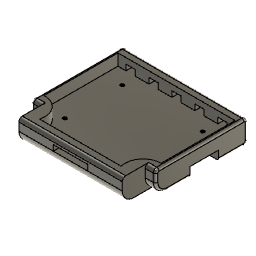
Carcasa Muñeca v2.2 (Autodesk Fusion 360 design; units mm, degrees)
Autodesk Fusion 360 part; units mm, degrees
sketch "Sketch10" plane through (0, 0, 0) normal (0, 0, 1) x (1, 0, 0)
  line L0 (0, -50) -> (0, 50) construction
  line L1 (0, 50) -> (-57, 50)
  line L2 (-57, 50) -> (-57, 0)
  line L3 (0, -50) -> (-45, -50)
  line L4 (-45, -50) -> (-45, -30)
  arc A0 (-57, 0) -> (-45, -30) centre (-7.0663, 2.5735) ccw
  line L5 (0, -50) -> (45, -50)
  line L6 (45, -50) -> (45, -30)
  arc A1 (45, -30) -> (57, 0) centre (7.0663, 2.5735) ccw
  line L7 (57, 50) -> (57, 0)
  line L8 (0, 50) -> (57, 50)
  dimension "d19" = 100
  dimension "d20" = 57
  dimension "d21" = 50
  dimension "d22" = 45
  dimension "d23" = 20
  dimension "d24" = 50
  dimension "d25" = 30
  constraint vertical L0
  constraint midpoint L0 origin
  constraint perpendicular L0 L1
  constraint perpendicular L1 L2
  constraint perpendicular L0 L3
  constraint perpendicular L3 L4
  constraint symmetric L3.start L0 L5.start
  constraint symmetric L1.start L0 L8.start
  constraint symmetric L0 L1.end L7.start
  constraint symmetric L0 L2.end A1.end
  constraint symmetric L0 L3.end L5.end
  constraint symmetric L0 L4.end L6.end
  constraint symmetric L0 A0 A1
  measures "d19" distance of L0.start L0.end
  measures "d20" distance of L0.end L1.end
  measures "d21" distance of L1.end L2.end
  measures "d22" distance of L0.start L3.end
  measures "d23" distance of L3.end L4.end
  measures "d24" radius of A0
  measures "d25" vertical distance of L2.end L4.end
sketch "Sketch12" plane through (0, 0, 0) normal (1, 0, 0) x (0, 1, 0)
  line L0 (0, 10) -> (0, -10) construction
  line L1 (0, 10) -> (47, 10)
  line L2 (50, 7) -> (50, -7)
  line L3 (47, -10) -> (0, -10)
  arc A0 (50, 7) -> (47, 10) centre (47, 7) ccw
  line L4 (0, 10) -> (-47, 10)
  line L5 (-50, 7) -> (-50, 0)
  line L6 (-40, -10) -> (0, -10)
  arc A1 (-47, 10) -> (-50, 7) centre (-47, 7) ccw
  arc A2 (-50, 0) -> (-40, -10) centre (-40, 0) ccw
  arc A3 (47, -10) -> (50, -7) centre (47, -7) ccw
  dimension "d30" = 3
  dimension "d31" = 47
  dimension "d34" = 3
  dimension "d35" = 10
  dimension "d36" = 7
  dimension "d37" = 40
  dimension "d38" = 3
  dimension "d39" = 47
  dimension "d40" = 14
  constraint vertical L0
  constraint midpoint L0 origin
  constraint perpendicular L0 L1
  constraint perpendicular L1 L2
  constraint tangent L1 A0
  constraint tangent L2 A0
  constraint perpendicular L0 L4
  constraint perpendicular L4 L5
  constraint tangent L5 A1
  constraint tangent L4 A1
  constraint tangent L6 A2
  constraint tangent L5 A2
  constraint tangent L3 A3
  constraint tangent L2 A3
  measures "d30" radius of A0
  measures "d31" distance of L0.start L1.end
  measures "d34" radius of A1
  measures "d35" radius of A2
  measures "d36" distance of L5.start L5.end
  measures "d37" distance of L0.end L6.start
  measures "d38" radius of A3
  measures "d39" distance of L0.end L3.start
  measures "d40" distance of L2.start L2.end
extrude "Extrude1" add sketch "Sketch12" along normal mid plane 90 makes body 1
ref_plane "PlanoDeObra18" through (-54, 0, 0) normal (-1, 0, 0) x (0, -1, 0)
sketch "Boceto31" plane through (-45, 0, 0) normal (-1, 0, 0) x (0, -1, 0)
  line L0 (47, 10) -> (-47, 10)
  arc A0 (-47, 10) -> (-50, 7) centre (-47, 7) ccw
  line L1 (-50, 7) -> (-50, -7)
  arc A1 (-50, -7) -> (-47, -10) centre (-47, -7) ccw
  line L2 (-47, -10) -> (0, -10)
  line L3 (0, -10) -> (40, -10)
  arc A2 (40, -10) -> (50, 0) centre (40, 0) ccw
  line L4 (50, 0) -> (50, 7)
  arc A3 (50, 7) -> (47, 10) centre (47, 7) ccw
  arc A4 (-50, -7) -> (-47, -10) centre (-47, -7) ccw
  line L5 (-47, -7) -> (-50, -7) construction
  line L6 (-47, -7) -> (-47, -10) construction
  line L7 (-47, -10) -> (20, -10)
  line L8 (-47, 10) -> (27, 10)
  line L9 (-50, 7) -> (-50, -7)
  arc A5 (30, 7) -> (26.9876, 10) centre (27, 7) ccw
  line L10 (27, 7) -> (30, 7) construction
  line L11 (27, 7) -> (26.9876, 10) construction
  arc A6 (20, -10) -> (30, 0) centre (20, 0) ccw
  line L12 (20, 0) -> (20, -10) construction
  line L13 (20, 0) -> (30, 0) construction
  line L14 (30, 0) -> (30, 7)
  dimension "d172" = 3
  dimension "d174" = 67
  dimension "d175" = 74
  dimension "d176" = 3
  dimension "d178" = 10
  constraint coincident A1.centre A4.centre
  constraint coincident A1.end L2.start
  constraint perpendicular L6 L7
  constraint coincident L0.end A0.start
  constraint parallel L0 L8
  constraint coincident A0.end L1.start
  constraint tangent A4 L9
  constraint tangent L8 A5
  constraint tangent L7 A6
  constraint tangent A6 L14
  constraint tangent A5 L14
  constraint perpendicular L8 L14
  measures "d172" radius of A4
  measures "d174" distance of A1.end L7.end
  measures "d175" distance of L0.end L8.end
  measures "d176" radius of A5
  measures "d178" radius of A6
extrude "Extruir14" add sketch "Boceto31" along normal blind 9 contours L0 A0 L1 A1 L2 L3 A4 L7 L8 L9 A5 A6 L14 bodies 1
sketch "Boceto32" plane through (45, 0, 0) normal (1, 0, 0) x (0, 1, 0)
  line L0 (47, 10) -> (-47, 10)
  arc A0 (-47, 10) -> (-50, 7) centre (-47, 7) ccw
  line L1 (-50, 7) -> (-50, 0)
  arc A1 (-50, 0) -> (-40, -10) centre (-40, 0) ccw
  line L2 (-40, -10) -> (0, -10)
  line L3 (0, -10) -> (47, -10)
  arc A2 (47, -10) -> (50, -7) centre (47, -7) ccw
  line L4 (50, -7) -> (50, 7)
  arc A3 (50, 7) -> (47, 10) centre (47, 7) ccw
  arc A4 (50, 7) -> (47, 10) centre (47, 7) ccw
  line L5 (47, 7) -> (50, 7) construction
  line L6 (47, 7) -> (47, 10) construction
  line L7 (47, 10) -> (-27, 10)
  arc A5 (47, -10) -> (50, -7) centre (47, -7) ccw
  line L8 (47, -7) -> (47, -10) construction
  line L9 (47, -7) -> (50, -7) construction
  line L10 (50, 7) -> (50, -7)
  line L11 (47, -10) -> (-20, -10)
  arc A6 (-30, 0) -> (-20, -10) centre (-20, 0) ccw
  line L12 (-20, 0) -> (-30, 0) construction
  line L13 (-20, 0) -> (-20, -10) construction
  arc A7 (-27, 10) -> (-30, 7) centre (-27, 7) ccw
  line L14 (-27, 7) -> (-27, 10) construction
  line L15 (-27, 7) -> (-30, 7) construction
  line L16 (-30, 7) -> (-30, 0)
  dimension "d182" = 3
  dimension "d184" = 74
  dimension "d185" = 3
  dimension "d187" = 67
  dimension "d188" = 10
  dimension "d190" = 3
  constraint coincident A3.centre A4.centre
  constraint coincident L0.start A3.end
  constraint perpendicular L6 L7
  constraint coincident A2.centre A5.centre
  constraint coincident L3.end A2.start
  constraint tangent A2 L10
  constraint perpendicular L10 L11
  constraint tangent A6 L16
  constraint tangent L7 A7
  constraint tangent L11 A6
  constraint tangent A5 L11
  constraint perpendicular L7 L16
  measures "d182" radius of A4
  measures "d184" distance of L0.start L7.end
  measures "d185" radius of A5
  measures "d187" distance of L3.end L11.end
  measures "d188" radius of A6
  measures "d190" radius of A7
extrude "Extruir15" add sketch "Boceto32" along normal blind 9 contours L0 L2 L3 A2 L4 A3 A4 L7 A5 L10 L11 A6 A7 L16 bodies 1
ref_plane "PlanoDeObra19" through (0, 0, 0) normal (0, 0, 1) x (0, -1, 0)
sketch "Boceto33" plane through (0, 0, 0) normal (0, 0, 1) x (1, 0, 0)
  line L0 (-43.8537, 42.0783) -> (51, 42.2395)
  line L1 (51, 42.2395) -> (-51, 42.2395)
  line L2 (-51, 42.2395) -> (-51, -22.125)
  line L3 (51, -22.125) -> (51, 42.2395)
  line L4 (-35.1587, -41.7605) -> (35.8108, -41.7605)
  arc A0 (-35.1587, -41.7605) -> (-51, -22.125) centre (-50.3046, -37.7717) ccw
  arc A1 (51, -22.125) -> (35.8108, -41.7605) centre (50.9606, -37.7871) ccw
  line L5 (0, 42.2395) -> (0.326, -41.7605)
  line L6 (54, -20) -> (54, 47)
  line L7 (-54, 47) -> (-54, -20)
  dimension "d202" = 84
  dimension "d256" = 3
  dimension "d257" = 3
  constraint horizontal L1
  constraint vertical L2
  constraint vertical L3
  constraint horizontal L4
  constraint equal L2 L3
  constraint equal A0 A1
  constraint midpoint L1 L5.start
  constraint midpoint L4 L5.end
  measures "d202" vertical distance of L5.start L5.end
  measures "d256" distance of L3 L6
  measures "d257" distance of L2 L7
extrude "Extruir16" cut sketch "Boceto33" along normal blind 10 bodies 1
ref_plane "PlanoDeObra20" through (54, 10, 10) normal (-1, 0, 0) x (0, -1, 0)
sketch "Boceto34" plane through (54, 10, 10) normal (-1, 0, 0) x (0, 0, -1)
  line L0 (20.0665, 10.0967) -> (12.0665, 10.0967)
  line L1 (12.0665, 10.0967) -> (12.0665, -14.9033)
  line L2 (12.0665, -14.9033) -> (20.0665, -14.9033)
  line L3 (20.0665, -14.9033) -> (20.0665, 10.0967)
  dimension "d205" = 8
  dimension "d206" = 25
  constraint horizontal L0
  constraint vertical L1
  constraint horizontal L2
  constraint vertical L3
  measures "d205" distance of L0.start L0.end
  measures "d206" distance of L0.start L2.end
extrude "Extruir17" cut sketch "Boceto34" along normal blind 15 bodies 1
ref_plane "PlanoDeObra21" through (46.5, -0.0967, -6.0333) normal (0, 1, 0) x (0, 0, -1)
sketch "Boceto35" plane through (46.5, -0.0967, -6.0333) normal (0, 1, 0) x (1, 0, 0)
  circle A0 centre (0, 0) radius 1.5
  dimension "d210" = 3
  constraint coincident A0.centre origin
  measures "d210" diameter of A0
extrude "Extruir18" add sketch "Boceto35" along normal up to surface (25 mm away) bodies 1
ref_plane "PlanoDeObra22" through (-54, 10, 0) normal (-1, 0, 0) x (0, -1, 0)
ref_plane "PlanoDeObra23" through (0, 50, 0) normal (0, 1, 0) x (0, 0, 1)
ref_plane "PlanoDeObra25" through (0, -50, 3.5) normal (0, -1, 0) x (0, 0, -1)
sketch "Boceto36" plane through (0, -50, 3.5) normal (0, -1, 0) x (1, 0, 0)
  line L0 (-15, 1.5) -> (15, 1.5)
  line L1 (15, 1.5) -> (15, -3.5)
  line L2 (15, -3.5) -> (-15, -3.5)
  line L3 (-15, -3.5) -> (-15, 1.5)
  line L4 (-15, 1.5) -> (15, -3.5) construction
  line L5 (15, 1.5) -> (-15, -3.5) construction
  point P0 (0, -1)
  dimension "d217" = 30
  dimension "d218" = 5
  constraint horizontal L0
  constraint perpendicular L0 L1
  constraint parallel L0 L2
  constraint parallel L1 L3
  constraint coincident L4 P0
  constraint coincident L5 P0
  measures "d217" distance of L1.end L2.end
  measures "d218" distance of L0.end L1.end
extrude "Extruir19" cut sketch "Boceto36" against normal blind 8.2397 bodies 1
fillet "Empalme5" radius 2 8 edges at (-54, 50, 0) (-54, 49.1213, -9.1213) (-54, 13.5, -10) (-54, -27.0711, -7.0711) (-54, -30, 3.5) (-54, -29.1213, 9.1213) (-54, 10, 10) (-54, 49.1213, 9.1213) on bodies 1
fillet "Empalme6" radius 2 9 edges at (54, 35.9516, -10) (54, 49.1213, -9.1213) (54, 50, 0) (54, 49.1213, 9.1213) (54, 10, 10) (54, -29.1213, 9.1213) (54, -30, 3.5) (54, -27.0711, -7.0711) (54, -10.0484, -10) on bodies 1
sketch "Boceto37" plane through (-54, 10, 0) normal (-1, 0, 0) x (0, 0, -1)
  line L0 (10.1981, 9.9042) -> (2.1981, 9.9042)
  line L1 (2.1981, 9.9042) -> (2.1981, -15.0958)
  line L2 (2.1981, -15.0958) -> (10.1981, -15.0958)
  line L3 (10.1981, -15.0958) -> (10.1981, 9.9042)
  dimension "d225" = 8
  dimension "d226" = 25
  constraint horizontal L0
  constraint vertical L1
  constraint horizontal L2
  constraint vertical L3
  measures "d225" distance of L0.start L0.end
  measures "d226" distance of L0.start L2.end
extrude "Extruir20" cut sketch "Boceto37" against normal blind 15 bodies 1
ref_plane "PlanoDeObra26" through (-46.5, 0.0958, -6.099) normal (0, 1, 0) x (0, 0, 1)
sketch "Boceto38" plane through (-46.5, 0.0958, -6.099) normal (0, 1, 0) x (1, 0, 0)
  circle A0 centre (0, 0) radius 1.5
  dimension "d233" = 3
  constraint coincident A0.centre origin
  measures "d233" diameter of A0
extrude "Extruir21" add sketch "Boceto38" along normal up to surface (25 mm away) bodies 1
sketch "Boceto39" plane through (0, 50, 0) normal (0, 1, 0) x (1, 0, 0)
  line L0 (44, 0) -> (36, 0)
  line L1 (36, 0) -> (36, -5)
  line L2 (36, -5) -> (44, -5)
  line L3 (44, -5) -> (44, 0)
  line L4 (52, 7) -> (52, -7)
  line L5 (24, 0) -> (16, 0)
  line L6 (16, 0) -> (16, -5)
  line L7 (16, -5) -> (24, -5)
  line L8 (24, -5) -> (24, 0)
  line L9 (4, 0) -> (-4, 0)
  line L10 (-4, 0) -> (-4, -5)
  line L11 (-4, -5) -> (4, -5)
  line L12 (4, -5) -> (4, 0)
  line L13 (11, -12) -> (-1, -12)
  line L14 (-16, 0) -> (-24, 0)
  line L15 (-24, 0) -> (-24, -5)
  line L16 (-24, -5) -> (-16, -5)
  line L17 (-16, -5) -> (-16, 0)
  line L18 (-36, 0) -> (-44, 0)
  line L19 (-44, 0) -> (-44, -5)
  line L20 (-44, -5) -> (-36, -5)
  line L21 (-36, -5) -> (-36, 0)
  line L22 (-52, -7) -> (-52, 7)
  dimension "d236" = 8
  dimension "d237" = 5
  dimension "d238" = 8
  dimension "d239" = 8
  dimension "d240" = 5
  dimension "d241" = 12
  dimension "d242" = 8
  dimension "d243" = 5
  dimension "d244" = 12
  dimension "d245" = 8
  dimension "d246" = 5
  dimension "d247" = 12
  dimension "d248" = 8
  dimension "d249" = 5
  dimension "d250" = 12
  dimension "d253" = 8
  constraint horizontal L0
  constraint vertical L1
  constraint horizontal L2
  constraint vertical L3
  constraint horizontal L5
  constraint vertical L6
  constraint horizontal L7
  constraint vertical L8
  constraint horizontal L9
  constraint vertical L10
  constraint horizontal L11
  constraint vertical L12
  constraint horizontal L13
  constraint horizontal L14
  constraint vertical L15
  constraint horizontal L16
  constraint vertical L17
  constraint horizontal L18
  constraint vertical L19
  constraint horizontal L20
  constraint vertical L21
  measures "d236" distance of L0.start L0.end
  measures "d237" distance of L0.start L2.end
  measures "d238" distance of L0.start L4
  measures "d239" distance of L5.start L5.end
  measures "d240" distance of L5.start L7.end
  measures "d241" distance of L0.end L5.start
  measures "d242" distance of L9.start L9.end
  measures "d243" distance of L9.start L11.end
  measures "d244" distance of L5.end L9.start
  measures "d245" distance of L14.start L14.end
  measures "d246" distance of L14.start L16.end
  measures "d247" distance of L9.end L14.start
  measures "d248" distance of L18.start L18.end
  measures "d249" distance of L18.start L20.end
  measures "d250" distance of L14.end L18.start
  measures "d253" distance of L18.end L22
extrude "Extruir22" cut sketch "Boceto39" against normal blind 8 bodies 1
sketch "Boceto40" plane through (0, 0, 0) normal (0, 0, 1) x (-1, 0, 0)
  line L0 (4, -42.2395) -> (16, -42.2395)
  line L1 (16, -42.2395) -> (16, -50)
  line L2 (16, -50) -> (24, -50)
  line L3 (24, -50) -> (24, -42.2395)
  line L4 (24, -42.2395) -> (36, -42.2395)
  line L5 (36, -42.2395) -> (36, -50)
  line L6 (36, -50) -> (44, -50)
  line L7 (44, -50) -> (44, -42.2395)
  line L8 (44, -42.2395) -> (51, -42.2395)
  line L9 (51, -42.2395) -> (51, 22.125)
  arc A0 (35.1587, 41.7605) -> (51, 22.125) centre (50.3046, 37.7717) ccw
  line L10 (35.1587, 41.7605) -> (15, 41.7605)
  line L11 (15, 41.7605) -> (15, 50)
  line L12 (15, 50) -> (-15, 50)
  line L13 (-15, 50) -> (-15, 41.7605)
  line L14 (-15, 41.7605) -> (-35.8108, 41.7605)
  arc A1 (-51, 22.125) -> (-35.8108, 41.7605) centre (-50.9606, 37.7871) ccw
  line L15 (-51, 22.125) -> (-51, -42.2395)
  line L16 (-51, -42.2395) -> (-44, -42.2395)
  line L17 (-44, -42.2395) -> (-44, -50)
  line L18 (-44, -50) -> (-36, -50)
  line L19 (-36, -50) -> (-36, -42.2395)
  line L20 (-36, -42.2395) -> (-24, -42.2395)
  line L21 (-24, -42.2395) -> (-24, -50)
  line L22 (-24, -50) -> (-16, -50)
  line L23 (-16, -50) -> (-16, -42.2395)
  line L24 (-16, -42.2395) -> (-4, -42.2395)
  line L25 (-4, -42.2395) -> (-4, -50)
  line L26 (-4, -50) -> (4, -50)
  line L27 (4, -50) -> (4, -42.2395)
sketch "Boceto41" plane through (0, 0, 0) normal (0, 0, 1) x (1, 0, 0)
  circle A0 centre (-35, 30) radius 1.525
  circle A1 centre (-35, -20) radius 1.525
  circle A2 centre (35, 30) radius 1.525
  circle A3 centre (35, -20) radius 1.525
  dimension "d260" = 3.05
  dimension "d261" = 3.05
  dimension "d262" = 3.05
  dimension "d264" = 70
  dimension "d265" = 50
  dimension "d266" = 3.05
  dimension "d267" = 70
  dimension "d268" = 50
  measures "d260" diameter of A0
  measures "d261" diameter of A1
  measures "d262" diameter of A2
  measures "d264" distance of A0.centre A2.centre
  measures "d265" distance of A0.centre A1.centre
  measures "d266" diameter of A3
  measures "d267" distance of A1.centre A3.centre
  measures "d268" distance of A2.centre A3.centre
extrude "Extruir23" cut sketch "Boceto41" against normal blind 5 bodies 1
move_body "Desplazar4" bodies 1 to x (1, 0, 0) y (0, 1, 0) z (0, 0, 1) at (12.846, -1.2909, -14.1369)
copy_body "Cuerpo - > Comp.2" bodies 1 removing the originals makes body 2 in component "Component'"
thread "Thread1" "ISO Metric profile 3.0 M3x0.5 6H" major diameter 3.086 minor diameter 2.529 pitch 0.5 angle 60 modelled right hand crest width 0.1368 on face at (47.3603, 27.2635, -17.4702) crest through (49.1105, 28.7091, -14.2619) on face at (47.808, -19.7664, -17.4702) crest through (49.1105, -21.2909, -14.2619) on face at (-20.721, 29.2307, -17.4702) crest through (-20.8895, 28.7091, -14.2619) on face at (-20.6309, -21.3669, -17.4702) crest through (-20.8895, -21.2909, -14.2619) on bodies 2 in component "Component'"
component "Component'" placed x (1, 0, 0) y (0, 1, 0) z (0, 0, 1) at (0, 0, 0)
